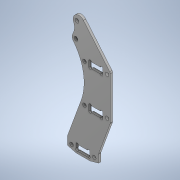
# Autodesk Inventor part: Head_vertical_frame_01
Saved by Autodesk Inventor 2020.4 (Build 244396000, 396)
## iProperties
Created: 2021-09-02
Part Number: Head_vertical_frame_01
Material: CFRP
Document SubType Name: Modeling
Designer: Masato
Density: 1.43 g/cm^3
Appearance: 滑らか - 標準の灰色
Mass: 6.2736 g
Surface Area: 52.8266 cm^2
Volume: 4.38713 cm^3
Author: Masato
Autodesk Inventor part; units mm, degrees
ref_plane "YZ Plane" through (0, 0, 0) normal (1, 0, 0) x (0, 1, 0)
ref_plane "XZ Plane" through (0, 0, 0) normal (0, 1, 0) x (-1, 0, 0)
ref_plane "XY Plane" through (0, 0, 0) normal (0, 0, 1) x (1, 0, 0)
sketch "スケッチ1" plane through (0, 0, 0) normal (0, 0, 1) x (1, 0, 0)
  line L0 (0, 0) -> (27, 0) construction
  line L1 (27, 0) -> (27, 5) construction
  line L2 (27, 5) -> (0, 5) construction
  line L3 (0, 5) -> (0, 0) construction
  line L4 (0, 2.5) -> (27, 2.5) construction
  line L5 (13.5, 5) -> (13.5, 0) construction
  circle A0 centre (3.7, 2.5) radius 1.55
  line L6 (7.5, 5) -> (7.5, 0) construction
  circle A1 centre (23.3, 2.5) radius 1.55
  line L7 (19.5, 5) -> (19.5, 0) construction
  line L8 (7.49, 5.01) -> (9.59, 5.01) construction
  line L9 (19.51, 5.01) -> (19.51, -0.01)
  line L10 (19.51, -0.01) -> (7.49, -0.01)
  line L11 (7.49, -0.01) -> (7.49, 5.01)
  line L12 (7.49, 5.01) -> (19.51, -0.01) construction
  line L13 (19.51, 5.01) -> (7.49, -0.01) construction
  line L14 (0, 0) -> (7.5, -2)
  line L15 (7.5, -2) -> (19.5, -2)
  line L16 (27, 0) -> (19.5, -2)
  arc A2 (9.59, 5.01) -> (7.49, 5.01) centre (8.54, 5.01) ccw
  arc A3 (19.51, 5.01) -> (17.41, 5.01) centre (18.46, 5.01) ccw
  line L17 (9.59, 5.01) -> (17.41, 5.01)
  line L18 (9.59, -0.01) -> (7.49, -0.01)
  line L19 (17.41, 5.01) -> (19.51, 5.01) construction
  line L20 (27, 7) -> (0, 7) construction
  line L21 (0, 0) -> (0, 7)
  line L22 (12.1912, 35) -> (37.1912, 35) construction
  line L23 (37.1912, 35) -> (37.1912, 40) construction
  line L24 (37.1912, 40) -> (12.1912, 40) construction
  line L25 (12.1912, 40) -> (12.1912, 35) construction
  line L26 (12.1912, 37.5) -> (37.1912, 37.5) construction
  line L27 (24.6912, 40) -> (24.6912, 35) construction
  circle A4 centre (14.8912, 37.5) radius 1.55
  line L28 (18.6912, 40) -> (18.6912, 35) construction
  line L29 (30.6912, 40) -> (30.6912, 35) construction
  circle A5 centre (34.4912, 37.5) radius 1.55
  line L30 (18.6812, 40.01) -> (20.7812, 40.01) construction
  line L31 (30.7012, 40.01) -> (30.7012, 34.99)
  line L32 (30.7012, 34.99) -> (28.6012, 34.99) construction
  line L33 (18.6812, 34.99) -> (18.6812, 40.01)
  line L34 (18.6812, 40.01) -> (30.7012, 34.99) construction
  line L35 (30.7012, 40.01) -> (18.6812, 34.99) construction
  arc A6 (20.7812, 40.01) -> (18.6812, 40.01) centre (19.7312, 40.01) ccw
  arc A7 (18.6812, 34.99) -> (20.7812, 34.99) centre (19.7312, 34.99) ccw
  arc A8 (30.7012, 40.01) -> (28.6012, 40.01) centre (29.6512, 40.01) ccw
  arc A9 (28.6012, 34.99) -> (30.7012, 34.99) centre (29.6512, 34.99) ccw
  line L36 (20.7812, 40.01) -> (28.6012, 40.01)
  line L37 (20.7812, 34.99) -> (18.6812, 34.99) construction
  line L38 (28.6012, 40.01) -> (30.7012, 40.01) construction
  line L39 (28.6012, 34.99) -> (20.7812, 34.99)
  line L40 (12.1912, 73) -> (12.1912, 68) construction
  circle A10 centre (14.8912, 70.5) radius 1.55
  line L41 (37.1912, 68) -> (37.1912, 73) construction
  line L42 (30.6912, 73) -> (30.6912, 68) construction
  circle A11 centre (34.4912, 70.5) radius 1.55
  line L43 (30.7012, 73.01) -> (30.7012, 67.99)
  line L44 (18.6912, 73) -> (18.6912, 68) construction
  line L45 (12.1912, 68) -> (37.1912, 68) construction
  line L46 (37.1912, 73) -> (12.1912, 73) construction
  line L47 (12.1912, 70.5) -> (37.1912, 70.5) construction
  line L48 (24.6912, 73) -> (24.6912, 68) construction
  line L49 (20.7812, 73.01) -> (28.6012, 73.01)
  line L50 (28.6012, 67.99) -> (20.7812, 67.99)
  line L51 (18.6812, 73.01) -> (30.7012, 67.99) construction
  line L52 (30.7012, 73.01) -> (18.6812, 67.99) construction
  arc A12 (30.7012, 73.01) -> (28.6012, 73.01) centre (29.6512, 73.01) ccw
  line L53 (28.6012, 73.01) -> (30.7012, 73.01) construction
  arc A13 (28.6012, 67.99) -> (30.7012, 67.99) centre (29.6512, 67.99) ccw
  line L54 (30.7012, 67.99) -> (28.6012, 67.99) construction
  line L55 (18.6812, 73.01) -> (20.7812, 73.01) construction
  line L56 (20.7812, 67.99) -> (18.6812, 67.99) construction
  arc A14 (20.7812, 73.01) -> (18.6812, 73.01) centre (19.7312, 73.01) ccw
  arc A15 (18.6812, 67.99) -> (20.7812, 67.99) centre (19.7312, 67.99) ccw
  line L57 (18.6812, 67.99) -> (18.6812, 73.01)
  line L58 (27, 0) -> (27, 6.6473)
  line L59 (37.1912, 35) -> (27.1206, 7.3314)
  line L60 (11.8992, 39.6929) -> (0, 7)
  line L61 (37.1912, 35) -> (37.1912, 73)
  line L62 (6.8054, 101.4338) -> (6.7491, 101.3865)
  arc A16 (4.7394, 86.3065) -> (5.3203, 95.7003) centre (-4.8938, 91.617) ccw
  circle A17 centre (-4.8938, 91.617) radius 14.6063 construction
  line L63 (1.0459, 61.9185) -> (-21.5815, 84.5459) construction
  line L64 (-21.5815, 84.5459) -> (-18.0459, 88.0815) construction
  line L65 (-18.0459, 88.0815) -> (4.5815, 65.4541) construction
  line L66 (4.5815, 65.4541) -> (1.0459, 61.9185) construction
  line L67 (1.0459, 61.9185) -> (-18.0459, 88.0815) construction
  line L68 (-21.5815, 84.5459) -> (4.5815, 65.4541) construction
  line L69 (13.8495, 100.8175) -> (37.1912, 73)
  arc A18 (11.8992, 39.6929) -> (5.2055, 80.7796) centre (-28.1256, 54.2607) ccw
  arc A19 (8.344, 97.7899) -> (6.2953, 101.0057) centre (-4.8938, 91.617) ccw construction
  arc A20 (5.0756, 80.942) -> (7.4988, 83.886) centre (-4.8938, 91.617) ccw construction
  circle A21 centre (8.344, 97.7899) radius 1.65
  circle A22 centre (7.4988, 83.886) radius 1.65
  arc A23 (13.8495, 100.8175) -> (6.8054, 101.4338) centre (10.0193, 97.6035) ccw
  arc A24 (6.7491, 101.3865) -> (5.3203, 95.7003) centre (9.9631, 97.5563) ccw
  arc A25 (4.7394, 86.3065) -> (5.2055, 80.7796) centre (9.1182, 83.8926) ccw
  arc A26 (27.1206, 7.3314) -> (27, 6.6473) centre (29, 6.6473) ccw
  arc A27 (7.49, 1.4749) -> (8.9749, -0.01) centre (8.2325, 0.7325) ccw
  arc A28 (18.0251, -0.01) -> (19.51, 1.4749) centre (18.7675, 0.7325) ccw
  point P0 (13.5, 2.5)
  point P1 (24.6912, 37.5)
  point P2 (24.6912, 70.5)
  point P3 (10.6356, 104.6477)
  point P4 (3.5327, 98.6877)
  point P5 (-8.5, 75)
  point P6 (19.51, 1.4749)
  point P7 (18.0251, -0.01)
  dimension "d0" = 27
  dimension "d1" = 5
  dimension "d2" = 3.1
  dimension "d3" = 12
  dimension "d4" = 19.6
  dimension "d5" = 0.01
  dimension "d6" = 0.01
  dimension "d7" = 2
  dimension "d8" = 12
  dimension "d9" = 1.05
  dimension "d10" = 7
  dimension "d11" = 25
  dimension "d12" = 5
  dimension "d13" = 3.1
  dimension "d14" = 12
  dimension "d15" = 19.6
  dimension "d16" = 0.01
  dimension "d17" = 0.01
  dimension "d20" = 1.05
  dimension "d22" = 25
  dimension "d23" = 5
  dimension "d24" = 3.1
  dimension "d25" = 12
  dimension "d26" = 19.6
  dimension "d27" = 0.01
  dimension "d28" = 0.01
  dimension "d29" = 1.05
  dimension "d30" = 70
  dimension "d31" = 66
  dimension "d32" = 33
  dimension "d37" = 5
  dimension "d38" = 75
  dimension "d39" = 135
  dimension "d40" = 8.5
  dimension "d46" = 11.8
  dimension "d47" = 32
  dimension "d48" = 50
  dimension "d49" = 6.8
  dimension "d50" = 11
  dimension "d51" = 29.2126
  dimension "d54" = 15
  dimension "d55" = 15
  dimension "d56" = 3.3
  dimension "d57" = 3.3
  dimension "d60" = 5
  dimension "d61" = 2
  dimension "d62" = 1.05
  constraints: 140 end point, 48 point on circle, 37 parallel, 29 centre point, 28 symmetric about line, 26 midpoint, 20 point on line, 18 perpendicular, 14 horizontal, 9 tangent, 4 equal radius, 3 coincident, 1 collinear, 1 line through centre, 1 vertical, 12 other
  measures "d0" distance of L2.end L1.end
  measures "d1" distance of L1.end L0.end
  measures "d2" diameter of A0
  measures "d3" distance of L7.end L6.end
  measures "d4" distance of A1.centre A0.centre
  measures "d5" horizontal distance of L6.start L8.start
  measures "d6" distance from line of L8 L6.start
  measures "d7" vertical distance of L14.end L0.start
  measures "d8" distance of L14.end L15.end
  measures "d9" radius of A2
  measures "d10" distance of L0.start L20.end
  measures "d11" distance of L25.start L23.end
  measures "d12" distance of L23.end L23.start
  measures "d13" diameter of A4
  measures "d14" distance of L29.end L28.end
  measures "d15" distance of A5.centre A4.centre
  measures "d16" horizontal distance of L28.start L34.start
  measures "d17" distance from line of L30 L28.start
  measures "d20" radius of A6
  measures "d22" distance of L46.start L46.end
  measures "d23" distance of L46.start L45.end
  measures "d24" diameter of A10
  measures "d25" distance of L42.end L44.end
  measures "d26" distance of A11.centre A10.centre
  measures "d27" horizontal distance of L44.start L57.end
  measures "d28" distance from line of L55 L44.start
  measures "d29" radius of A14
  measures "d30" angle of L20 L59
  measures "d31" vertical distance of L46.start L20.start
  measures "d32" vertical distance of L20.start L23.end
  measures "d37" distance of L63.end L64.end
  measures "d38" vertical distance of point (-8.5, 75) L0.start
  measures "d39" angle of L63 L3
  measures "d40" horizontal distance of L0.start point (-8.5, 75)
  measures "d46" distance from line of A17.centre L65
  measures "d47" distance of L63.start L63.end
  measures "d48" angle of L0 L69
  measures "d49" distance from line of A16.centre L64
  measures "d50" radius of A16
  measures "d51" diameter of A17
  measures "d56" diameter of A21
  measures "d57" diameter of A22
  measures "d60" radius of A23
  measures "d61" radius of A26
  measures "d62" radius of A27
extrude "押し出し1" add sketch "スケッチ1" against normal blind 2
fillet "フィレット1" radius 2 5 edges at (37.1912, 73, -1) (37.1912, 35, -1) (0, 7, -1) (7.5, -2, -1) (19.5, -2, -1)
equation "\"d5\" = d6"
equation "\"d12\" = d1"
equation "\"d13\" = d2"
equation "\"d14\" = d3"
equation "\"d15\" = d4"
equation "\"d16\" = d6"
equation "\"d17\" = d6"
equation "\"d22\" = d11"
equation "\"d23\" = d1"
equation "\"d24\" = d2"
equation "\"d25\" = d3"
equation "\"d26\" = d4"
equation "\"d27\" = d6"
equation "\"d28\" = d6"
equation "\"d32\" = 0.5 * d31"
